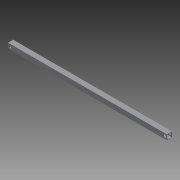
# Autodesk Inventor part: Long Bar
Saved by Autodesk Inventor 2015 (Build 190159000, 159)
## iProperties
Created: 2016-01-11
Part Number: Long Bar
Material: Generic
Document SubType Name: Modeling
Designer: Applegate
Density: 1 g/cm^3
Appearance: Default
Author: Applegate
Autodesk Inventor part; units mm, degrees
ref_plane "YZ Plane" through (0, 0, 0) normal (1, 0, 0) x (0, 1, 0)
ref_plane "XZ Plane" through (0, 0, 0) normal (0, 1, 0) x (-1, 0, 0)
ref_plane "XY Plane" through (0, 0, 0) normal (0, 0, 1) x (1, 0, 0)
sketch "Sketch1" plane through (0, 0, 0) normal (1, 0, 0) x (0, 1, 0)
  line L0 (-12.7, 12.7) -> (12.7, 12.7)
  line L1 (12.7, 12.7) -> (12.7, -12.7)
  line L2 (12.7, -12.7) -> (-12.7, -12.7)
  line L3 (-12.7, -12.7) -> (-12.7, 12.7)
  line L4 (-11.1125, 11.1125) -> (11.1125, 11.1125)
  line L5 (11.1125, 11.1125) -> (11.1125, -10.8514)
  line L6 (11.1125, -10.8514) -> (-11.1125, -10.8514)
  line L7 (-11.1125, -10.8514) -> (-11.1125, 11.1125)
  point P0 (0, 0)
  point P1 (0, 12.7)
  point P2 (-12.7, 0)
  dimension "d0" = 25.4
  dimension "d1" = 25.4
  dimension "d2" = 1.5875
  dimension "d3" = 1.5875
  dimension "d4" = 1.5875
  constraints: 16 end point, 4 parallel, 2 horizontal, 2 midpoint, 2 perpendicular, 1 horizontal alignment, 1 vertical alignment
  measures "d0" distance of L0.start L0.end
  measures "d1" distance of L2.end L0.start
  measures "d2" horizontal distance of L4.start L0.start
  measures "d3" horizontal distance of L2.end L6.end
  measures "d4" horizontal distance of L0.end L4.end
extrude "Extrusion1" add sketch "Sketch1" along normal blind 787.4
sketch "Sketch2" plane through (0, -12.7, 12.7) normal (0, 0, 1) x (1, 0, 0)
  circle A0 centre (9.525, 12.7) radius 6.35
  circle A1 centre (777.875, 12.7) radius 6.35
  line L0 (787.4, 25.4) -> (787.4, 0) projected
  point P0 (0, 12.7)
  dimension "d7" = 12.7
  dimension "d8" = 9.525
  dimension "d9" = 12.7
  dimension "d10" = 9.525
  constraints: 2 centre point
  measures "d7" diameter of A0
  measures "d8" distance of A0.centre point (0, 12.7)
  measures "d9" diameter of A1
  measures "d10" distance from line of A1.centre L0
extrude "Extrusion2" cut sketch "Sketch2" against normal blind 50.8
equation "\"d1\" = d0"
equation "\"d3\" = d2"
equation "\"d4\" = d2"
equation "\"d9\" = d7"
equation "\"d10\" = d8"
body "Solid1"
